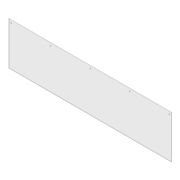
# Autodesk Inventor part: FE-00010
Saved by Autodesk Inventor 2012 (Build 160160000, 160)
## iProperties
Created: 2008-06-02
Part Number: FE-00010
Document SubType Name: Modeling
Designer: mcyr
Density: 1 g/cm^3
Description: Field Plastic "C"
Mass: 5602.11 g
Surface Area: 17947.5 cm^2
Volume: 5602.11 cm^3
Material: Default
Title: FE-00010
Author: mcyr
Autodesk Inventor part; units mm, degrees
ref_plane "YZ Plane" through (0, 0, 0) normal (1, 0, 0) x (0, 1, 0)
ref_plane "XZ Plane" through (0, 0, 0) normal (0, 1, 0) x (-1, 0, 0)
ref_plane "XY Plane" through (0, 0, 0) normal (0, 0, 1) x (1, 0, 0)
sketch "Sketch1" plane through (0, 0, 0) normal (0, 0, 1) x (1, 0, 0)
  line L0 (-44.6869, 0.2846) -> (1784.1131, 0.2846)
  line L1 (1784.1131, 482.8846) -> (-44.6869, 482.8846)
  line L2 (-44.6869, 482.8846) -> (-44.6869, 0.2846)
  line L3 (1784.1131, 0.2846) -> (1784.1131, 482.8846)
  circle A0 centre (-19.2869, 451.1346) radius 4.7625
  circle A1 centre (425.2131, 451.1346) radius 4.7625
  circle A2 centre (869.7131, 451.1346) radius 4.7625
  circle A3 centre (1314.2131, 451.1346) radius 4.7625
  circle A4 centre (1758.7131, 451.1346) radius 4.7625
  dimension "d0" = 482.6
  dimension "d1" = 1828.8
  dimension "d7" = 25.4
  dimension "d8" = 469.9
  dimension "d9" = 914.4
  dimension "d10" = 1358.9
  dimension "d11" = 1803.4
  dimension "d12" = 31.75
  dimension "d13" = 31.75
  dimension "d14" = 31.75
  dimension "d15" = 31.75
  dimension "d16" = 31.75
  dimension "d19" = 9.525
  dimension "d20" = 9.525
  dimension "d21" = 9.525
  dimension "d22" = 9.525
  dimension "d23" = 9.525
  constraints: 8 end point, 5 centre point, 2 parallel, 1 horizontal, 1 perpendicular
  measures "d0" distance of L1.end L0.start
  measures "d1" distance of L0.start L0.end
  measures "d7" horizontal distance of A0.centre L1.end
  measures "d8" horizontal distance of A1.centre L1.end
  measures "d9" horizontal distance of A2.centre L1.end
  measures "d10" horizontal distance of A3.centre L1.end
  measures "d11" horizontal distance of A4.centre L1.end
  measures "d12" vertical distance of L1.end A0.centre
  measures "d13" distance from line of L1 A1.centre
  measures "d14" distance from line of L1 A2.centre
  measures "d15" distance from line of L1 A3.centre
  measures "d16" distance from line of L1 A4.centre
  measures "d19" diameter of A0
  measures "d20" diameter of A1
  measures "d21" diameter of A2
  measures "d22" diameter of A3
  measures "d23" diameter of A4
extrude "Extrusion1" add sketch "Sketch1" along normal blind 6.35
body "Solid1"
